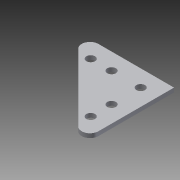
# Autodesk Inventor part: Chassis Corner Plate V1.500
Saved by Autodesk Inventor 2013 (Build 170138000, 138)
## iProperties
Created: 2013-01-13
Part Number: Chassis Corner Plate V1.500
Material: Aluminum 6061
Document SubType Name: Modeling
Designer: Moses
Mass: 20.6104 g
Surface Area: 58.1202 cm^2
Volume: 7.60532 cm^3
Density: 2.71 g/cm^3
Author: Moses
Autodesk Inventor part; units mm, degrees
ref_plane "YZ Plane" through (0, 0, 0) normal (1, 0, 0) x (0, 1, 0)
ref_plane "XZ Plane" through (0, 0, 0) normal (0, 1, 0) x (-1, 0, 0)
ref_plane "XY Plane" through (0, 0, 0) normal (0, 0, 1) x (1, 0, 0)
sketch "Sketch1" plane through (0, 0, 0) normal (0, 1, 0) x (-1, 0, 0)
  line L0 (0, 0) -> (73.025, 0)
  line L1 (0, 0) -> (0, 73.025)
  line L2 (0, 73.025) -> (73.025, 0)
  line L3 (12.7, 0) -> (12.7, 60.325) construction
  line L4 (0, 12.7) -> (60.325, 12.7) construction
  circle A0 centre (12.7, 34.925) radius 3.302
  circle A1 centre (34.925, 12.7) radius 3.302
  circle A2 centre (50.8, 12.7) radius 3.302
  circle A3 centre (12.7, 50.8) radius 3.302
  circle A4 centre (12.7, 12.7) radius 3.302
  line L5 (0, 34.925) -> (38.1, 34.925) construction
  line L6 (34.925, 38.1) -> (34.925, 0) construction
  dimension "d0" = 73.025
  dimension "d1" = 73.025
  dimension "d2" = 12.7
  dimension "d3" = 12.7
  dimension "d4" = 6.604
  dimension "d5" = 6.604
  dimension "d6" = 6.604
  dimension "d7" = 6.604
  dimension "d8" = 15.875
  dimension "d9" = 15.875
  dimension "d10" = 6.604
  dimension "d14" = 34.925
  dimension "d15" = 34.925
  constraints: 16 point on line, 14 end point, 5 centre point, 3 perpendicular, 1 horizontal, 1 parallel
  measures "d0" distance of L0.start L0.end
  measures "d1" distance of L0.start L1.end
  measures "d2" distance between parallel lines of L0 L4
  measures "d3" distance between parallel lines of L3 L1
  measures "d4" diameter of A0
  measures "d5" diameter of A1
  measures "d6" diameter of A2
  measures "d7" diameter of A3
  measures "d8" distance of A0.centre A3.centre
  measures "d9" distance of A2.centre A1.centre
  measures "d10" diameter of A4
  measures "d14" distance between parallel lines of L6 L1
  measures "d15" distance between parallel lines of L0 L5
extrude "Extrusion1" add sketch "Sketch1" along normal blind 3.175
fillet "Fillet1" radius 6.35 2 edges at (0, 1.5875, 73.025) (-73.025, 1.5875, 0)
equation "\"d0\" = d1"
equation "\"d2\" = d3"
equation "\"d4\" = d7"
equation "\"d5\" = d7"
equation "\"d6\" = d7"
equation "\"d9\" = d8"
equation "\"d10\" = d7"
equation "\"d15\" = d14"
body "Solid1"
